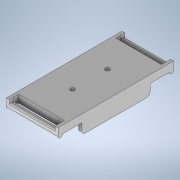
# Autodesk Inventor part: Battery_holder_2
Saved by Autodesk Inventor 2022 (Build 260153000, 153)
## iProperties
Created: 2023-02-02
Part Number: Battery_holder_2
Material: Generic
Document SubType Name: Modeling
Designer: scott
Density: 1 g/cm^3
Appearance: Default
Author: scott
Autodesk Inventor part; units mm, degrees
ref_plane "YZ Plane" through (0, 0, 0) normal (1, 0, 0) x (0, 1, 0)
ref_plane "XZ Plane" through (0, 0, 0) normal (0, 1, 0) x (-1, 0, 0)
ref_plane "XY Plane" through (0, 0, 0) normal (0, 0, 1) x (1, 0, 0)
sketch "Sketch1" plane through (0, 0, 0) normal (0, 1, 0) x (-1, 0, 0)
  line L0 (15, 30) -> (-15, 30)
  line L1 (-15, 30) -> (-15, -30)
  line L2 (-15, -30) -> (15, -30)
  line L3 (15, -30) -> (15, 30)
  line L4 (0, 11.5) -> (-15, 11.5)
  line L5 (-15, 11.5) -> (-15, -11.5)
  line L6 (-15, -11.5) -> (0, -11.5)
  line L7 (0, -11.5) -> (0, 11.5)
  point P0 (0, 0)
  dimension "d0" = 30
  dimension "d1" = 60
  dimension "d2" = 30
  dimension "d3" = 15
  dimension "d4" = 23
  dimension "d5" = 18.5
  constraints: 16 end point, 4 parallel, 2 horizontal, 2 perpendicular, 1 point on line
  measures "d0" distance of L1.end L2.end
  measures "d1" distance of L0.end L1.end
  measures "d2" distance from line of point (0, 0) L2
  measures "d3" distance from line of L1 point (0, 0)
  measures "d4" distance of L6.end L4.start
  measures "d5" distance between parallel lines of L4 L0
extrude "Extrusion1" add sketch "Sketch1" along normal blind 2
hole "Hole1" at (0, 0, -11.5) at (0, 0, 11.5) direction (0, 1, 0) diameter 2.8 end through all counterbore diameter 5 counterbore depth 0.5
sketch "Sketch2" plane through (0, 0, 0) normal (0, -1, 0) x (1, 0, 0)
  line L0 (17, 32) -> (-17, 32)
  line L1 (-17, 32) -> (-17, -32)
  line L2 (-17, -32) -> (17, -32)
  line L3 (17, -32) -> (17, 32)
  line L4 (15, 30) -> (15, -30) projected
  line L5 (-15, -30) -> (-15, 30) projected
  line L6 (15, 30) -> (-15, 30)
  line L7 (-15, 30) -> (-15, -30)
  line L8 (-15, -30) -> (15, -30)
  line L9 (15, -30) -> (15, 30)
  point P0 (0, 0)
  point P1 (-15, 30)
  dimension "d15" = 34
  dimension "d16" = 64
  dimension "d17" = 32
  dimension "d18" = 17
  constraints: 16 end point, 4 parallel, 2 horizontal, 2 perpendicular
  measures "d15" distance of L1.end L2.end
  measures "d16" distance of L0.end L1.end
  measures "d17" distance from line of point (0, 0) L2
  measures "d18" distance from line of point (0, 0) L1
extrude "Extrusion2" add sketch "Sketch2" along normal blind 3 and the other way blind 2
sketch "Sketch3" plane through (-17, -3, -32) normal (-1, 0, 0) x (0, 0, 1)
  line L0 (2, 0) -> (62, 0) projected
  line L1 (54.5, 0) -> (9.5, 0)
  line L2 (9.5, 0) -> (9.5, -7)
  line L3 (9.5, -7) -> (54.5, -7)
  line L4 (54.5, -7) -> (54.5, 0)
  line L5 (2, 3) -> (62, 3) projected
  line L6 (64, 0) -> (64, 5) projected
  circle A0 centre (52, -4.5) radius 2.5
  circle A1 centre (12, -4.5) radius 2.5
  point P0 (32, 3)
  point P1 (52, -7)
  point P2 (54.5, -4.5)
  point P3 (9.5, 0)
  point P4 (9.5, -4.5)
  point P5 (12, -7)
  dimension "d23" = 10
  dimension "d24" = 45
  dimension "d25" = 9.5
  dimension "d26" = 5
  dimension "d27" = 5
  dimension "d28" = 2.5
  dimension "d29" = 2.5
  constraints: 8 end point, 2 centre point, 2 parallel, 2 tangent, 1 horizontal, 1 perpendicular, 1 point on line
  measures "d23" distance between parallel lines of L5 L3
  measures "d24" distance of L2.end L3.end
  measures "d25" distance between parallel lines of L4 L6
  measures "d26" diameter of A0
  measures "d27" diameter of A1
  measures "d28" distance from line of L2 A1.centre
  measures "d29" distance from line of L4 A0.centre
extrude "Extrusion3" add sketch "Sketch3" against normal up to surface (2 mm away) contours L0 L4 A0 L3 A1 L2 | A1 | A0
mirror "Mirror1" about plane through (0, 0, 0) normal (1, 0, 0) of "Extrusion3"
sketch "Sketch6" plane through (0, -3, 0) normal (0, -1, 0) x (1, 0, 0)
  line L0 (15, 30) -> (-15, 30)
  line L1 (-15, 30) -> (-15, 35)
  line L2 (-15, 35) -> (15, 35)
  line L3 (15, 35) -> (15, 30)
  line L4 (17, 32) -> (-17, 32) projected
  line L5 (17, 32) -> (-17, 32)
  line L6 (-17, 32) -> (-17, 38)
  line L7 (-17, 38) -> (17, 38)
  line L8 (17, 38) -> (17, 32)
  point P0 (0, 0)
  point P1 (15, 32)
  point P2 (-15, 32)
  dimension "d34" = 3
  dimension "d35" = 6
  constraints: 16 end point, 4 parallel, 2 horizontal, 2 perpendicular
  measures "d34" distance between parallel lines of L2 L4
  measures "d35" distance of L5.end L6.end
extrude "Extrusion4" add sketch "Sketch6" against normal up to surface (5 mm away) contours L3 L2 L1 L4 L6 L7 L8
sketch "Sketch7" plane through (0, 2, 0) normal (0, 1, 0) x (1, 0, 0)
  line L0 (-15, -35) -> (15, -35) projected
  line L1 (17, -38) -> (-17, -38) projected
  line L2 (15, -35) -> (-14.9996, -35)
  line L3 (-14.9996, -35) -> (-14.9996, -38)
  line L4 (-14.9996, -38) -> (15, -38)
  line L5 (15, -38) -> (15, -35)
  point P0 (0, 0)
  constraints: 8 end point, 2 parallel, 1 horizontal, 1 perpendicular, 1 point on line
extrude "Extrusion5" cut sketch "Sketch7" against normal blind 2
sketch "Sketch8" plane through (-17, -3, -32) normal (-1, 0, 0) x (0, 0, 1)
  line L0 (70, 0) -> (54.5, 0) projected
  circle A0 centre (68.5, 0) radius 1.5
  point P0 (32, 3)
  point P1 (67, 0)
  dimension "d41" = 3
  constraints: 1 point on line, 3 other
extrude "Extrusion6" add sketch "Sketch8" against normal up to surface (34 mm away) contours A0 L0 picked at (68.5603, -0.4964)
mirror "Mirror2" about plane through (0, 0, 0) normal (0, 0, 1) of "Extrusion4", "Extrusion5", "Extrusion6"
fillet "Fillet2" radius 1 4 edges at (0.0002, 0, -38) (0.0002, 0, -35) (0.0002, 0, 38) (0.0002, 0, 35)
equation "\"d2\" = 0.5 * d1"
equation "\"d3\" = 0.5 * d0"
equation "\"d5\" = -0.5 * d4 + 0.5 * d1"
equation "\"d17\" = 0.5 * d16"
equation "\"d18\" = 0.5 * d15"
body "Solid1"
